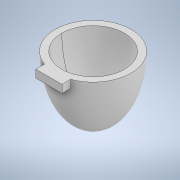
# Autodesk Inventor part: Egg
Saved by Autodesk Inventor 2022 (Build 260153000, 153)
## iProperties
Created: 2022-02-15
Part Number: Egg
Material: Generic
Document SubType Name: Modeling
Designer: Nathan Griffith
Density: 1 g/cm^3
Appearance: Default
Author: Nathan Griffith
Autodesk Inventor part; units mm, degrees
ref_plane "YZ Plane" through (0, 0, 0) normal (1, 0, 0) x (0, 1, 0)
ref_plane "XZ Plane" through (0, 0, 0) normal (0, 1, 0) x (-1, 0, 0)
ref_plane "XY Plane" through (0, 0, 0) normal (0, 0, 1) x (1, 0, 0)
sketch "Sketch1" plane through (0, 0, 0) normal (0, 0, 1) x (1, 0, 0)
  line L0 (0, 0) -> (0, 55.88)
  line L1 (-15.24, 55.88) -> (-30.48, 55.88)
  line L2 (-30.48, 55.88) -> (-30.48, 0)
  line L3 (0, 0) -> (-30.48, 0)
  line L4 (-15.24, 55.88) -> (-15.24, 0)
  line L5 (-15.24, 27.94) -> (-30.48, 27.94)
  ellipse E0 centre (-15.24, 27.94) end of major axis (-15.24, 55.88) minor radius 15.24 (-15.24, 55.88) -> (-15.24, 0) ccw
  dimension "d0" = 55.88
  dimension "d1" = 30.48
  dimension "d2" = 90
  constraints: 12 end point, 3 midpoint, 2 perpendicular, 2 vertical, 1 horizontal, 5 other
  measures "d0" distance of L0.start L0.end
  measures "d1" distance of L0.end L1.end
  measures "d2" angle of L1 L0
revolve "Revolution1" add sketch "Sketch1" angle 360 about axis through (-15.24, 55.88, 0) along (0, -1, 0) picked at (-18.3, 11.1925) contours L4 E0 L5
shell "Shell1" thickness 3.175 outward yes removed faces 1 at (-9.0238, 27.94, 3.6617)
sketch "Sketch2" plane through (-15.24, 27.94, 0) normal (0, 1, 0) x (1, 0, 0)
  line L0 (-6.35, -21.4741) -> (6.35, -21.4741)
  line L1 (6.35, -21.4741) -> (6.35, -13.8541)
  line L2 (6.35, -13.8541) -> (-6.35, -13.8541)
  line L3 (-6.35, -13.8541) -> (-6.35, -21.4741)
  circle A0 centre (0, 0) radius 18.415 projected
  circle A1 centre (0, 0) radius 15.24 projected
  point P0 (15.24, 0)
  point P1 (-18.415, 0)
  point P2 (-15.24, 0)
  dimension "d7" = 12.7
  dimension "d8" = 7.62
  constraints: 8 end point, 2 parallel, 2 point on circle, 1 horizontal, 1 horizontal alignment, 1 perpendicular
  measures "d7" distance of L2.end L1.end
  measures "d8" distance of L1.end L0.end
extrude "Extrusion1" add sketch "Sketch2" against normal blind 3.81 contours L3 A0 L1 L0 | L3 A1 L1 A0 picked at (-3.9186, -16.8211)
body "Solid1"
